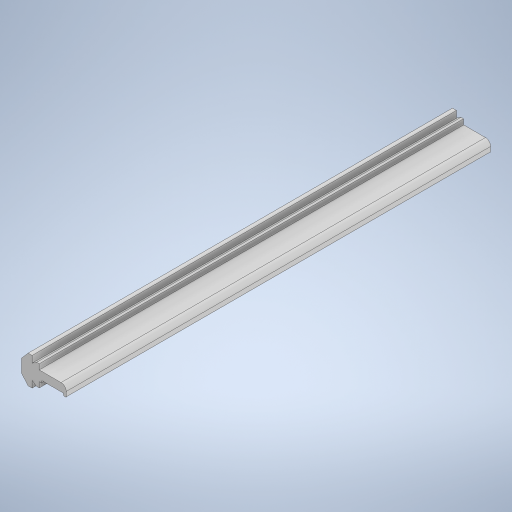
# Autodesk Inventor part: LED Strip Top Mount
Saved by Autodesk Inventor 2023 (Build 270158000, 158)
## iProperties
Created: 2024-01-21
Part Number: LED Strip Top Mount
Material: Generic
Document SubType Name: Modeling
Designer: Lyall
Density: 1 g/cm^3
Appearance: Default
Author: Lyall
Autodesk Inventor part; units mm, degrees
ref_plane "YZ Plane" through (0, 0, 0) normal (1, 0, 0) x (0, 1, 0)
ref_plane "XZ Plane" through (0, 0, 0) normal (0, 1, 0) x (-1, 0, 0)
ref_plane "XY Plane" through (0, 0, 0) normal (0, 0, 1) x (1, 0, 0)
sketch "Sketch1" plane through (0, 0, 0) normal (0, 0, 1) x (1, 0, 0)
  line L0 (0.0426, 8.3509) -> (2.1366, 8.3509) construction
  line L1 (-5.93, 6.5274) -> (-3.3043, 9.5646)
  line L2 (-3.3043, 9.5646) -> (-1.75, 9.5646)
  line L3 (-1.75, 9.5646) -> (-1.75, 6.9793)
  line L4 (-1.75, 6.9793) -> (0, 8.1293)
  line L5 (0, 8.1293) -> (0, 0)
  line L6 (0, 0) -> (-1.75, 1.15)
  line L7 (-1.75, 1.15) -> (-1.75, -1.4354)
  line L8 (-1.75, -1.4354) -> (-3.3043, -1.4354)
  line L9 (-3.3043, -1.4354) -> (-5.93, 1.6019)
  line L10 (-5.93, 1.6019) -> (-5.93, 6.5274)
  dimension "d16" = 0
  dimension "d17" = 0
  constraints: 22 end point, 1 horizontal
  measures "d16" distance of point (0, 0) L5.end
  measures "d17" distance of L5.end point (0, 0)
extrude "Extrusion1" add sketch "Sketch1" along normal blind 164.9
sketch "Sketch2" plane through (0, 0, 0) normal (1, 0, 0) x (0, 0, -1)
  line L0 (0, 8.1293) -> (-164.9, 8.1293) projected
  line L1 (0, 0) -> (0, 8.1293) projected
  line L2 (-164.9, 8.1293) -> (0, 8.1293)
  line L3 (0, 8.1293) -> (0, 0)
  line L4 (0, 0) -> (-164.9, 0)
  line L5 (-164.9, 0) -> (-164.9, 8.1293)
  constraints: 8 end point, 2 parallel, 1 horizontal, 1 perpendicular
extrude "Extrusion2" add sketch "Sketch2" along normal blind 1
sketch "Sketch3" plane through (1, 0, 0) normal (1, 0, 0) x (0, 0, -1)
  line L0 (-164.9, 8.1293) -> (-164.9, 0) projected
  line L1 (0, 2.065) -> (-164.9, 2.065)
  line L2 (-164.9, 2.065) -> (-164.9, 6.065)
  line L3 (-164.9, 6.065) -> (0, 6.065)
  line L4 (0, 6.065) -> (0, 2.065)
  line L5 (0, 2.065) -> (-164.9, 6.065) construction
  line L6 (-164.9, 2.065) -> (0, 6.065) construction
  line L7 (0, 0) -> (0, 8.1293) projected
  point P0 (-82.45, 4.065)
  dimension "d22" = 4
  dimension "d28" = 0
  constraints: 12 end point, 2 midpoint, 2 parallel, 1 horizontal, 1 perpendicular, 1 point on line
  measures "d22" distance of L1.end L2.end
  measures "d28" distance between parallel lines of L7 L4
extrude "Extrusion3" add sketch "Sketch3" along normal blind 10.5
sketch "Sketch4" plane through (1, 2.065, 0) normal (0, -1, 0) x (1, 0, 0)
  point P0 (-1, 0)
sketch "Sketch5" plane through (1, 2.065, 0) normal (0, -1, 0) x (1, 0, 0)
  line L0 (0, 164.9) -> (10.5, 164.9) projected
  line L1 (9.5, -0.1) -> (1, -0.1)
  line L2 (1, -0.1) -> (1, 164.9)
  line L3 (1, 164.9) -> (9.5, 164.9)
  line L4 (9.5, 164.9) -> (9.5, -0.1)
  line L5 (9.5, -0.1) -> (1, 164.9) construction
  line L6 (1, -0.1) -> (9.5, 164.9) construction
  point P0 (-1, 0)
  point P1 (5.25, 82.4)
  dimension "d25" = 8.5
  constraints: 12 end point, 2 midpoint, 2 parallel, 1 horizontal, 1 perpendicular, 1 point on line
  measures "d25" distance of L2.end L3.end
extrude "Extrusion4" cut sketch "Sketch5" against normal blind 0.9
fillet "Fillet1" radius 2 1 edges at (11.5, 6.065, 82.45)
fillet "Fillet2" radius 0.2 1 edges at (10.5, 2.965, 82.45)
fillet "Fillet3" radius 0.2 1 edges at (2, 2.965, 82.45)
fillet "Fillet4" radius 0.2 3 edges at (11.5, 2.065, 82.45) (10.5, 2.065, 82.45) (2, 2.065, 82.45)
body "Solid1"
